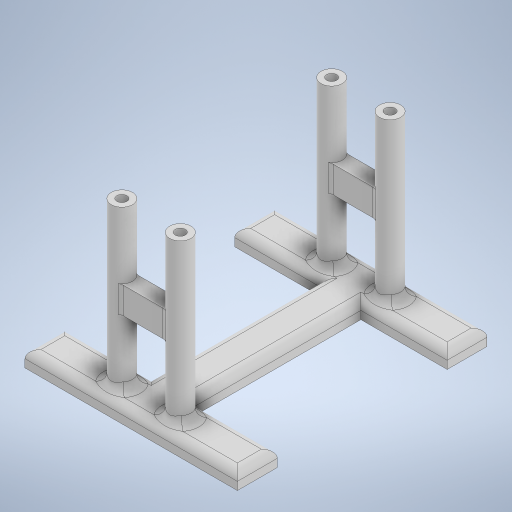
# Autodesk Inventor part: carrello
Saved by Autodesk Inventor 2023.2 (Build 272271030, 271C)
## iProperties
Created: 2023-11-28
Part Number: carrello
Material: Generic
Document SubType Name: Modeling
Designer: matti
Density: 1 g/cm^3
Appearance: Default
Author: matti
Autodesk Inventor part; units mm, degrees
ref_plane "XZ Plane" through (0, 0, 0) normal (0, 1, 0) x (-1, 0, 0)
ref_plane "XY Plane" through (0, 0, 0) normal (0, 0, 1) x (1, 0, 0)
sketch "Sketch1" plane through (0, 0, 0) normal (0, 1, 0) x (-1, 0, 0)
  line L0 (40, 47) -> (-40, 47)
  line L1 (-40, 47) -> (-40, 32)
  line L2 (-40, 32) -> (40, 32)
  line L3 (40, 32) -> (40, 47)
  line L4 (40, 39.5) -> (-40, 39.5) construction
  line L5 (0, -65.8) -> (0, 65.8) projected
  line L6 (75.7321, 0) -> (-79.5679, 0) construction
  line L7 (40, -47) -> (-40, -47)
  line L8 (-40, -47) -> (-40, -32)
  line L9 (-40, -32) -> (40, -32)
  line L10 (40, -32) -> (40, -47)
  line L11 (40, -39.5) -> (-40, -39.5) construction
  line L12 (0, 32) -> (7.5, 32)
  line L13 (7.5, 32) -> (7.5, -32)
  line L14 (0, -32) -> (-7.5, -32)
  line L15 (-7.5, -32) -> (-7.5, 32)
  point P0 (0, 0)
  dimension "d0" = 80
  dimension "d1" = 15
  dimension "d12" = 39.5
  dimension "d13" = 79
  dimension "d14" = 7.5
  dimension "d15" = 7.5
  constraints: 30 end point, 6 symmetric about line, 5 point on line, 4 midpoint, 3 perpendicular, 2 horizontal, 2 parallel, 1 other
  measures "d0" distance of L1.end L2.end
  measures "d1" distance of L2.end L0.start
  measures "d12" distance between parallel lines of L6 L4
  measures "d13" distance between parallel lines of L11 L4
  measures "d14" distance of L12.start L12.end
  measures "d15" distance of L14.start L14.end
extrude "Extrusion1" add sketch "Sketch1" along normal blind 6
fillet "Fillet1" radius 3 12 edges at (0, 6, 47) (40, 6, 39.5) (-23.75, 6, 32) (23.75, 6, 32) (-40, 6, 39.5) (23.75, 6, -32) (-23.75, 6, -32) (40, 6, -39.5) (0, 6, -47) (-40, 6, -39.5) (7.5, 6, 0) (-7.5, 6, 0)
sketch "Sketch2" plane through (0, 6, 0) normal (0, 1, 0) x (1, 0, 0)
  line L0 (-37, -35) -> (-4.5, -35) projected
  line L1 (-37, -44) -> (-37, -35) projected
  line L2 (37, -44) -> (-37, -44) projected
  line L3 (37, -35) -> (37, -44) projected
  line L4 (-37, -44) -> (-37, -35) construction
  line L5 (-37, -39.5) -> (37, -39.5) construction
  line L6 (37, -35) -> (37, -44) construction
  line L7 (-37, -35) -> (37, -35) construction
  line L8 (0, -35) -> (0, -44) construction
  circle A0 centre (-11, -39.5) radius 4
  circle A1 centre (11, -39.5) radius 4
  line L9 (0, 65.8) -> (0, -65.8) construction
  line L10 (4.5, -35) -> (37, -35) projected
  line L11 (37, 35) -> (4.5, 35) projected
  line L12 (37, 44) -> (37, 35) projected
  line L13 (-37, 44) -> (37, 44) projected
  line L14 (-37, 35) -> (-37, 44) projected
  line L15 (-4.5, 35) -> (-37, 35) projected
  line L16 (-4.5, -35) -> (-4.5, 35) projected
  line L17 (4.5, 35) -> (4.5, -35) projected
  line L18 (-56, 0) -> (56, 0) projected
  circle A2 centre (-11, 39.5) radius 4
  circle A3 centre (11, 39.5) radius 4
  point P0 (0, 0)
  dimension "d5" = 8
  dimension "d6" = 22
  constraints: 4 centre point, 4 end point, 4 midpoint, 3 symmetric about line, 1 perpendicular, 1 point on line, 4 other
  measures "d5" diameter of A0
  measures "d6" distance of A1.centre A0.centre
extrude "Extrusion2" add sketch "Sketch2" along normal blind 60 contours A0 | A1 | A2 | A3
fillet "Fillet2" radius 3 4 edges at (-15, 6, 39.5) (7, 6, 39.5) (7, 6, -39.5) (-15, 6, -39.5)
sketch "Sketch3" plane through (-11, 66, 39.5) normal (0, 1, 0) x (1, 0, 0)
  circle A0 centre (0, 0) radius 1.875
  circle A1 centre (22, 0) radius 4 projected
  circle A2 centre (22, 0) radius 1.875
  line L0 (-45, 39.5) -> (67, 39.5) projected
  circle A3 centre (0, 79) radius 1.875
  circle A4 centre (22, 79) radius 1.875
  point P0 (11, 39.5)
  dimension "d10" = 3.75
  dimension "d11" = 3.75
  constraints: 4 centre point, 2 symmetric about line, 1 coincident, 2 other
  measures "d10" diameter of A0
  measures "d11" diameter of A2
extrude "Extrusion3" cut sketch "Sketch3" against normal blind 6 contours A0 | A2 | A3 | A4
ref_plane "Work Plane1" through (11, 0, 0) normal (1, 0, 0) x (0, 1, 0)
sketch "Sketch4" plane through (11, 0, 0) normal (1, 0, 0) x (0, 1, 0)
  line L0 (41, -42.5) -> (31, -42.5)
  line L1 (31, -42.5) -> (31, -36.5)
  line L2 (31, -36.5) -> (41, -36.5)
  line L3 (41, -36.5) -> (41, -42.5)
  line L4 (120.1597, -39.5) -> (56.9301, -39.5) construction
  line L5 (6, 35) -> (6, -35) projected
  line L6 (8.4544, -35.5) -> (66, -35.5) projected
  line L7 (8.4544, -43.5) -> (66, -43.5) projected
  point P0 (0, 0)
  point P1 (31, -39.5)
  dimension "d19" = 6
  dimension "d20" = 10
  dimension "d21" = 25
  dimension "d23" = 1
  constraints: 10 end point, 2 horizontal, 2 parallel, 1 midpoint, 1 perpendicular, 1 other
  measures "d19" distance of L2.end L0.start
  measures "d20" distance of L1.end L2.end
  measures "d21" distance from line of L5 point (31, -39.5)
  measures "d23" distance between parallel lines of L7 L0
extrude "Extrusion4" add sketch "Sketch4" against normal blind 22
fillet "Fillet3" radius 3 4 edges at (8.3542, 36, -42.5) (-8.3542, 36, -42.5) (-8.3542, 36, -36.5) (8.3542, 36, -36.5)
mirror "Mirror1" about plane through (0, 0, 0) normal (0, 0, 1)
body "Solid1"
